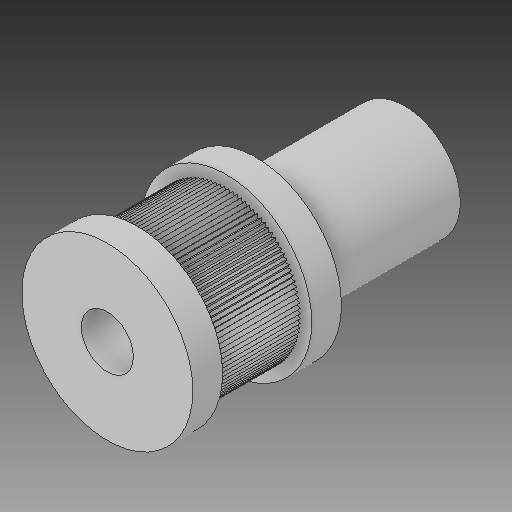
# Autodesk Inventor part: Faja motor
Saved by Autodesk Inventor 2019 (Build 230136000, 136)
## iProperties
Created: 2020-02-04
Part Number: Faja motor
Material: Generic
Document SubType Name: Modeling
Designer: Elías Sánchez
Density: 1 g/cm^3
Appearance: Default
Description: Impresión 3D
Author: Elías Sánchez
Autodesk Inventor part; units mm, degrees
ref_plane "YZ Plane" through (0, 0, 0) normal (1, 0, 0) x (0, 1, 0)
ref_plane "XZ Plane" through (0, 0, 0) normal (0, 1, 0) x (-1, 0, 0)
sketch "Sketch1" plane through (0, 0, 0) normal (0, 0, 1) x (1, 0, 0)
  circle A0 centre (0, 0) radius 10
  dimension "d0" = 20
  constraints: 1 centre point, 1 coincident
  measures "d0" diameter of A0
extrude "Extrusion1" add sketch "Sketch1" along normal blind 20
sketch "Sketch2" plane through (0, 0, 20) normal (0, 0, 1) x (1, 0, 0)
  circle A0 centre (0, 0) radius 10 projected
  line L0 (0, -14) -> (0, 14) projected
  circle A1 centre (0, 0) radius 9.4958
  line L1 (0, 9.4958) -> (-0.2887, 9.9958)
  line L2 (0, 9.4958) -> (0.2887, 9.9958)
  dimension "d9" = 30
  dimension "d10" = 30
  dimension "d11" = 0.5
  dimension "d12" = 0.5
  constraints: 4 end point, 2 point on circle, 1 coincident, 1 vertical alignment, 2 other
  measures "d9" angle of L0 L1
  measures "d10" angle of L0 L2
  measures "d11" vertical distance of L1.start L1.end
  measures "d12" vertical distance of L1.start L2.end
extrude "Extrusion2" cut sketch "Sketch2" against normal blind 20 contours L2 L0 A0 | L0 L1 A0
pattern_circular "Circular Pattern1" count 108 over 360 about axis through (0, 0, 0) along (0, 0, 1) of "Extrusion2"
sketch "Sketch3" plane through (0, 0, 20) normal (0, 0, 1) x (1, 0, 0)
  circle A0 centre (0, 0) radius 11.5
  dimension "d18" = 23
  constraints: 1 centre point, 1 coincident
  measures "d18" diameter of A0
extrude "Extrusion3" add sketch "Sketch3" against normal blind 4
ref_plane "Work Plane1" through (0, 0, 10) normal (0, 0, 1) x (1, 0, 0)
mirror "Mirror1" about plane through (0, 0, 10) normal (0, 0, 1) of "Extrusion3"
sketch "Sketch5" plane through (0, 0, 0) normal (0, 0, -1) x (-1, 0, 0)
  circle A0 centre (0, 0) radius 7.5
  dimension "d25" = 15
  constraints: 1 centre point, 1 coincident
  measures "d25" diameter of A0
extrude "Extrusion5" add sketch "Sketch5" along normal blind 20
sketch "Sketch4" plane through (0, 0, 20) normal (0, 0, 1) x (1, 0, 0)
  circle A0 centre (0, 0) radius 3.5
  dimension "d22" = 7
  constraints: 1 centre point, 1 coincident
  measures "d22" diameter of A0
extrude "Extrusion4" cut sketch "Sketch4" against normal blind 40
equation "\"d10\" = d9"
equation "\"d12\" = d11"
body "Solid1"
